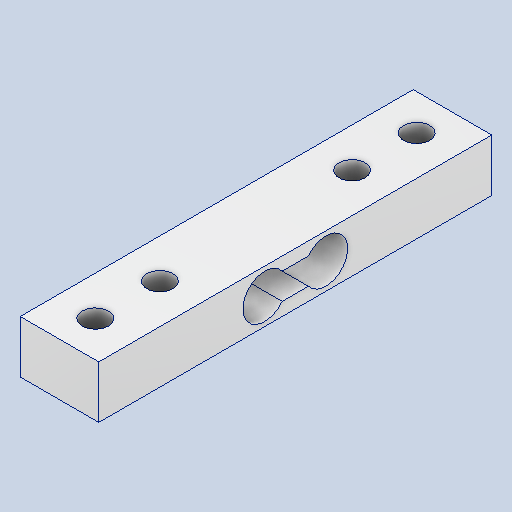
# Autodesk Inventor part: load_cell_SC616C
Saved by Autodesk Inventor 2025 (Build 290162000, 162)
## iProperties
Created: 2025-09-02
Part Number: load_cell_SC616C
Material: アルミニウム 6061
Document SubType Name: Modeling
Designer: sooo1
Density: 2.7 g/cm^3
Appearance: アルミニウム - フラット
Author: sooo1
Autodesk Inventor part; units mm, degrees
ref_plane "YZ Plane" through (0, 0, 0) normal (1, 0, 0) x (0, 1, 0)
ref_plane "XZ Plane" through (0, 0, 0) normal (0, 1, 0) x (-1, 0, 0)
ref_plane "XY Plane" through (0, 0, 0) normal (0, 0, 1) x (1, 0, 0)
sketch "スケッチ1" plane through (0, 0, 0) normal (0, 1, 0) x (-1, 0, 0)
  line L0 (4.5, 22.5) -> (-4.5, 22.5)
  line L1 (-4.5, 22.5) -> (-4.5, -22.5)
  line L2 (-4.5, -22.5) -> (4.5, -22.5)
  line L3 (4.5, -22.5) -> (4.5, 22.5)
  line L4 (4.5, 22.5) -> (-4.5, -22.5) construction
  line L5 (-4.5, 22.5) -> (4.5, -22.5) construction
  line L6 (0, -31.5) -> (0, 31.5) construction
  line L7 (6.3, 0) -> (-6.3, 0) construction
  circle A0 centre (0, 11) radius 1.5
  circle A1 centre (0, 18.4) radius 1.5
  circle A2 centre (0, -11) radius 1.5
  circle A3 centre (0, -18.4) radius 1.5
  point P0 (0, 0)
  dimension "d0" = 45
  dimension "d1" = 9
  dimension "d2" = 3
  dimension "d3" = 22
  dimension "d4" = 7.4
  constraints: 12 end point, 4 centre point, 2 midpoint, 2 parallel, 2 point on line, 2 symmetric about line, 1 equal radius, 1 horizontal, 1 perpendicular, 2 other
  measures "d0" distance of L2.end L0.start
  measures "d1" distance of L0.start L0.end
  measures "d2" diameter of A0
  measures "d3" diameter of A0.centre L7
  measures "d4" distance of A1.centre A0.centre
extrude "押し出し1" add sketch "スケッチ1" along normal blind 6
sketch "スケッチ2" plane through (0, 0, 0) normal (1, 0, 0) x (0, 1, 0)
  line L0 (-1.2, 0) -> (7.2, 0) construction
  line L1 (0, -22.5) -> (0, 22.5) construction
  line L2 (0, 22.5) -> (6, 22.5) construction
  line L3 (6, -22.5) -> (6, 22.5) construction
  line L4 (0, -22.5) -> (6, -22.5) construction
  line L5 (3, 22.5) -> (3, -22.5) construction
  circle A0 centre (3, 3.5) radius 2.5
  circle A1 centre (3, -3.5) radius 2.5
  line L6 (4.5, 1.5) -> (4.5, -1.5)
  line L7 (1.5, 1.5) -> (1.5, -1.5)
  point P0 (0, 0)
  dimension "d7" = 5
  dimension "d8" = 7
  dimension "d9" = 3
  constraints: 6 end point, 3 symmetric about line, 2 midpoint, 1 horizontal, 1 point on line, 1 vertical, 6 other
  measures "d8" diameter of point (3, 3.5) L0
  measures "d9" diameter of L6 L5
extrude "押し出し2" cut sketch "スケッチ2" along normal through all both and the other way through all
